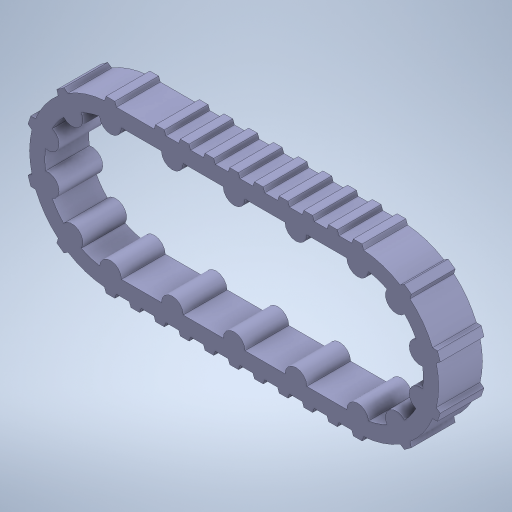
# Autodesk Inventor part: Guntas_Belt_New
Saved by Autodesk Inventor 2024 (Build 280153000, 153)
## iProperties
Created: 2023-07-07
Part Number: Guntas_Belt_New
Material: Generic
Document SubType Name: Modeling
Designer: manas
Density: 1 g/cm^3
Appearance: Slate Blue
Author: manas
Autodesk Inventor part; units mm, degrees
ref_plane "YZ Plane" through (0, 0, 0) normal (1, 0, 0) x (0, 1, 0)
ref_plane "XZ Plane" through (0, 0, 0) normal (0, 1, 0) x (-1, 0, 0)
ref_plane "XY Plane" through (0, 0, 0) normal (0, 0, 1) x (1, 0, 0)
sketch "Sketch1" plane through (0, 0, 0) normal (0, 0, 1) x (1, 0, 0)
  arc A0 (0, 75) -> (0, -75) centre (0, 0) ccw
  arc A1 (0, 92.5) -> (0, -92.5) centre (0, 0) ccw
  circle A2 centre (0, 75) radius 12.5
  circle A3 centre (-44.0839, 60.6763) radius 12.5
  circle A4 centre (-71.3292, 23.1763) radius 12.5
  circle A5 centre (-71.3292, -23.1763) radius 12.5
  circle A6 centre (-44.0839, -60.6763) radius 12.5
  circle A7 centre (0, -75) radius 12.5
  line L0 (0, 97.5) -> (-5, 97.5)
  line L1 (0, 97.5) -> (5, 97.5)
  line L2 (-5, 97.5) -> (-6.914, 92.2412)
  line L3 (-5, 97.5) -> (0.5963, 97.5) construction
  line L4 (5, 97.5) -> (6.914, 92.2412)
  line L5 (-57.3091, 78.8792) -> (-61.3541, 75.9402)
  line L6 (-61.3541, 75.9402) -> (-56.8267, 79.2296) construction
  line L7 (-57.3091, 78.8792) -> (-53.264, 81.8181)
  line L8 (-53.264, 81.8181) -> (-48.6245, 78.6887)
  line L9 (-61.3541, 75.9402) -> (-59.8116, 70.5608)
  line L10 (-92.728, 30.1292) -> (-94.2731, 25.3739)
  line L11 (-94.2731, 25.3739) -> (-92.5438, 30.6962) construction
  line L12 (-92.728, 30.1292) -> (-91.1829, 34.8844)
  line L13 (-91.1829, 34.8844) -> (-85.5901, 35.0797)
  line L14 (-94.2731, 25.3739) -> (-89.8632, 21.9285)
  line L15 (-92.728, -30.1292) -> (-91.1829, -34.8844)
  line L16 (-91.1829, -34.8844) -> (-92.9123, -29.5621) construction
  line L17 (-92.728, -30.1292) -> (-94.2731, -25.3739)
  line L18 (-94.2731, -25.3739) -> (-89.8632, -21.9285)
  line L19 (-91.1829, -34.8844) -> (-85.5901, -35.0797)
  line L20 (-57.3091, -78.8792) -> (-53.264, -81.8181)
  line L21 (-53.264, -81.8181) -> (-57.7914, -78.5287) construction
  line L22 (-57.3091, -78.8792) -> (-61.3541, -75.9402)
  line L23 (-61.3541, -75.9402) -> (-59.8116, -70.5608)
  line L24 (-53.264, -81.8181) -> (-48.6245, -78.6887)
  line L25 (0, -97.5) -> (5, -97.5)
  line L26 (5, -97.5) -> (-0.5963, -97.5) construction
  line L27 (0, -97.5) -> (-5, -97.5)
  line L28 (-5, -97.5) -> (-6.914, -92.2412)
  line L29 (5, -97.5) -> (6.914, -92.2412)
  line L30 (0, 92.5) -> (141.25, 92.5)
  line L31 (0, -92.5) -> (141.25, -92.5)
  line L32 (0, -92.5) -> (141.25, -92.5) construction
  line L33 (0, 75) -> (141.25, 75)
  line L34 (0, -75) -> (141.25, -75)
  line L35 (28.25, 97.5) -> (33.25, 97.5)
  line L36 (28.25, 97.5) -> (23.25, 97.5)
  line L37 (33.25, 97.5) -> (35.0699, 92.5)
  line L38 (23.25, 97.5) -> (21.4301, 92.5)
  line L39 (56.5, 97.5) -> (61.5, 97.5)
  line L40 (56.5, 97.5) -> (51.5, 97.5)
  line L41 (61.5, 97.5) -> (63.3199, 92.5)
  line L42 (51.5, 97.5) -> (49.6801, 92.5)
  line L43 (84.75, 97.5) -> (89.75, 97.5)
  line L44 (84.75, 97.5) -> (79.75, 97.5)
  line L45 (89.75, 97.5) -> (91.5699, 92.5)
  line L46 (79.75, 97.5) -> (77.9301, 92.5)
  line L47 (113, 97.5) -> (118, 97.5)
  line L48 (113, 97.5) -> (108, 97.5)
  line L49 (118, 97.5) -> (119.8199, 92.5)
  line L50 (108, 97.5) -> (106.1801, 92.5)
  line L51 (141.25, 97.5) -> (146.25, 97.5)
  line L52 (141.25, 97.5) -> (136.25, 97.5)
  line L53 (146.25, 97.5) -> (148.0699, 92.5)
  line L54 (136.25, 97.5) -> (134.4301, 92.5)
  circle A8 centre (70.625, 75) radius 12.5
  circle A9 centre (141.25, 75) radius 12.5
  line L55 (141.25, 92.5) -> (141.25, -92.5) construction
  line L56 (0, -92.5) -> (141.25, -92.5)
  line L57 (0, -75) -> (141.25, -75)
  line L58 (28.25, -97.5) -> (33.25, -97.5)
  line L59 (28.25, -97.5) -> (23.25, -97.5)
  line L60 (33.25, -97.5) -> (35.0699, -92.5)
  line L61 (23.25, -97.5) -> (21.4301, -92.5)
  line L62 (56.5, -97.5) -> (61.5, -97.5)
  line L63 (56.5, -97.5) -> (51.5, -97.5)
  line L64 (61.5, -97.5) -> (63.3199, -92.5)
  line L65 (51.5, -97.5) -> (49.6801, -92.5)
  line L66 (84.75, -97.5) -> (89.75, -97.5)
  line L67 (84.75, -97.5) -> (79.75, -97.5)
  line L68 (89.75, -97.5) -> (91.5699, -92.5)
  line L69 (79.75, -97.5) -> (77.9301, -92.5)
  line L70 (113, -97.5) -> (118, -97.5)
  line L71 (113, -97.5) -> (108, -97.5)
  line L72 (118, -97.5) -> (119.8199, -92.5)
  line L73 (108, -97.5) -> (106.1801, -92.5)
  line L74 (141.25, -97.5) -> (146.25, -97.5)
  line L75 (141.25, -97.5) -> (136.25, -97.5)
  line L76 (146.25, -97.5) -> (148.0699, -92.5)
  line L77 (136.25, -97.5) -> (134.4301, -92.5)
  circle A10 centre (70.625, -75) radius 12.5
  circle A11 centre (141.25, -75) radius 12.5
  line L78 (141.25, -92.5) -> (141.25, 92.5) construction
  arc A12 (282.5, -75) -> (282.5, 75) centre (282.5, 0) ccw
  arc A13 (282.5, -92.5) -> (282.5, 92.5) centre (282.5, 0) ccw
  circle A14 centre (282.5, 75) radius 12.5
  circle A15 centre (326.5839, 60.6763) radius 12.5
  circle A16 centre (353.8292, 23.1763) radius 12.5
  circle A17 centre (353.8292, -23.1763) radius 12.5
  circle A18 centre (326.5839, -60.6763) radius 12.5
  circle A19 centre (282.5, -75) radius 12.5
  line L79 (282.5, 97.5) -> (287.5, 97.5)
  line L80 (282.5, 97.5) -> (277.5, 97.5)
  line L81 (287.5, 97.5) -> (289.414, 92.2412)
  line L82 (287.5, 97.5) -> (281.9037, 97.5) construction
  line L83 (277.5, 97.5) -> (275.586, 92.2412)
  line L84 (339.8091, 78.8792) -> (343.8541, 75.9402)
  line L85 (343.8541, 75.9402) -> (339.3267, 79.2296) construction
  line L86 (339.8091, 78.8792) -> (335.764, 81.8181)
  line L87 (335.764, 81.8181) -> (331.1245, 78.6887)
  line L88 (343.8541, 75.9402) -> (342.3116, 70.5608)
  line L89 (375.228, 30.1292) -> (376.7731, 25.3739)
  line L90 (376.7731, 25.3739) -> (375.0438, 30.6962) construction
  line L91 (375.228, 30.1292) -> (373.6829, 34.8844)
  line L92 (373.6829, 34.8844) -> (368.0901, 35.0797)
  line L93 (376.7731, 25.3739) -> (372.3632, 21.9285)
  line L94 (375.228, -30.1292) -> (373.6829, -34.8844)
  line L95 (373.6829, -34.8844) -> (375.4123, -29.5621) construction
  line L96 (375.228, -30.1292) -> (376.7731, -25.3739)
  line L97 (376.7731, -25.3739) -> (372.3632, -21.9285)
  line L98 (373.6829, -34.8844) -> (368.0901, -35.0797)
  line L99 (339.8091, -78.8792) -> (335.764, -81.8181)
  line L100 (335.764, -81.8181) -> (340.2914, -78.5287) construction
  line L101 (339.8091, -78.8792) -> (343.8541, -75.9402)
  line L102 (343.8541, -75.9402) -> (342.3116, -70.5608)
  line L103 (335.764, -81.8181) -> (331.1245, -78.6887)
  line L104 (282.5, -97.5) -> (277.5, -97.5)
  line L105 (277.5, -97.5) -> (283.0963, -97.5) construction
  line L106 (282.5, -97.5) -> (287.5, -97.5)
  line L107 (287.5, -97.5) -> (289.414, -92.2412)
  line L108 (277.5, -97.5) -> (275.586, -92.2412)
  line L109 (282.5, 92.5) -> (141.25, 92.5)
  line L110 (282.5, -92.5) -> (141.25, -92.5)
  line L111 (282.5, -92.5) -> (141.25, -92.5) construction
  line L112 (282.5, 75) -> (141.25, 75)
  line L113 (282.5, -75) -> (141.25, -75)
  line L114 (254.25, 97.5) -> (249.25, 97.5)
  line L115 (254.25, 97.5) -> (259.25, 97.5)
  line L116 (249.25, 97.5) -> (247.4301, 92.5)
  line L117 (259.25, 97.5) -> (261.0699, 92.5)
  line L118 (226, 97.5) -> (221, 97.5)
  line L119 (226, 97.5) -> (231, 97.5)
  line L120 (221, 97.5) -> (219.1801, 92.5)
  line L121 (231, 97.5) -> (232.8199, 92.5)
  line L122 (197.75, 97.5) -> (192.75, 97.5)
  line L123 (197.75, 97.5) -> (202.75, 97.5)
  line L124 (192.75, 97.5) -> (190.9301, 92.5)
  line L125 (202.75, 97.5) -> (204.5699, 92.5)
  line L126 (169.5, 97.5) -> (164.5, 97.5)
  line L127 (169.5, 97.5) -> (174.5, 97.5)
  line L128 (164.5, 97.5) -> (162.6801, 92.5)
  line L129 (174.5, 97.5) -> (176.3199, 92.5)
  line L130 (141.25, 97.5) -> (136.25, 97.5)
  line L131 (141.25, 97.5) -> (146.25, 97.5)
  line L132 (136.25, 97.5) -> (134.4301, 92.5)
  line L133 (146.25, 97.5) -> (148.0699, 92.5)
  circle A20 centre (211.875, 75) radius 12.5
  circle A21 centre (141.25, 75) radius 12.5
  line L134 (282.5, -75) -> (141.25, -75)
  circle A22 centre (211.875, -75) radius 12.5
  line L135 (197.75, -97.5) -> (192.75, -97.5)
  line L136 (197.75, -97.5) -> (202.75, -97.5)
  line L137 (202.75, -97.5) -> (204.5699, -92.5)
  line L138 (282.5, -92.5) -> (141.25, -92.5)
  line L139 (259.25, -97.5) -> (261.0699, -92.5)
  line L140 (254.25, -97.5) -> (259.25, -97.5)
  line L141 (254.25, -97.5) -> (249.25, -97.5)
  line L142 (249.25, -97.5) -> (247.4301, -92.5)
  line L143 (221, -97.5) -> (219.1801, -92.5)
  line L144 (226, -97.5) -> (221, -97.5)
  line L145 (231, -97.5) -> (232.8199, -92.5)
  line L146 (226, -97.5) -> (231, -97.5)
  line L147 (169.5, -97.5) -> (164.5, -97.5)
  line L148 (169.5, -97.5) -> (174.5, -97.5)
  line L149 (164.5, -97.5) -> (162.6801, -92.5)
  line L150 (174.5, -97.5) -> (176.3199, -92.5)
  line L151 (192.75, -97.5) -> (190.9301, -92.5)
  line L152 (146.25, -97.5) -> (148.0699, -92.5)
  line L153 (141.25, -97.5) -> (146.25, -97.5)
  line L154 (141.25, -97.5) -> (136.25, -97.5)
  line L155 (136.25, -97.5) -> (134.4301, -92.5)
  circle A23 centre (141.25, -75) radius 12.5
  point P0 (270, -75)
  point P1 (224.375, -75)
  point P2 (199.375, -75)
  point P3 (153.75, -75)
  point P4 (128.75, -75)
  point P5 (83.125, -75)
  point P6 (58.125, -75)
  point P7 (12.5, -75)
  point P8 (-12.4565, -73.9583)
  point P9 (-33.3941, -67.1553)
  point P10 (-53.5492, -52.5118)
  point P11 (-66.4893, -34.7012)
  point P12 (-74.1878, -11.0075)
  point P13 (-74.1878, 11.0075)
  point P14 (-66.4893, 34.7012)
  point P15 (-53.5492, 52.5118)
  point P16 (-33.3941, 67.1553)
  point P17 (-12.4565, 73.9583)
  point P18 (12.5, 75)
  point P19 (58.125, 75)
  point P20 (83.125, 75)
  point P21 (128.75, 75)
  point P22 (153.75, 75)
  point P23 (199.375, 75)
  point P24 (224.375, 75)
  point P25 (270, 75)
  point P26 (294.9565, 73.9583)
  point P27 (315.8941, 67.1553)
  point P28 (336.0492, 52.5118)
  point P29 (348.9893, 34.7012)
  point P30 (356.6878, 11.0075)
  point P31 (356.6878, -11.0075)
  point P32 (348.9893, -34.7012)
  point P33 (336.0492, -52.5118)
  point P34 (315.8941, -67.1553)
  point P35 (294.9565, -73.9583)
  point P36 (6.8199, 92.5)
  point P37 (6.8199, -92.5)
  point P38 (275.6801, -92.5)
  point P39 (275.6801, 92.5)
  dimension "d5" = 180
  dimension "d13" = 180
  dimension "d29" = 28.25
  dimension "d38" = 70.625
  constraints: 312 end point, 98 symmetric about line, 24 centre point, 12 horizontal, 10 point on circle, 4 coincident, 4 midpoint, 4 point on line, 2 equal length, 1 tangent, 117 other
  measures "d29" distance of L36.end L40.end
  measures "d38" distance of A8.centre A9.centre
extrude "Extrusion1" add sketch "Sketch1" along normal mid plane 50 contours L33 A2 A0 | A0 A2 L33 | A3 A0 | A0 A3 | A8 L33 | L33 A8 | A4 A0 | A0 A4 | A9 L112 L33 | L33 L112 A9 | A5 A0 | A0 A5 | A20 L112 | L112 A20 | A6 A0 | A0 A6 | L112 A12 A14 | A14 A12 L112 | A7 L34 A0 | A0 L34 A7 | A15 A12 | A12 A15 | A10 L34 | L34 A10 | A16 A12 | A12 A16 | A11 L113 L34 | L34 L113 A11 | A17 A12 | A12 A17 | A22 L113 | L113 A22 | A18 A12 | A12 A18 | L113 A12 A19 | A19 A12 L113 | L30 L109 A13 L110 L31 A1 | A1 L2 L0 L1 L4 L30 | A1 L9 L5 L7 L8 | A1 L14 L10 L12 L13 | L42 L40 L39 L41 L30 | A1 L19 L15 L17 L18 | L46 L44 L43 L45 L30 | A1 L24 L20 L22 L23 | L50 L48 L47 L49 L30 | A1 L31 L29 L25 L27 L28 | L54 L52 L51 L53 L109 L30 | L31 L60 L58 L59 L61 | L128 L126 L127 L129 L109 | L31 L64 L62 L63 L65 | L124 L122 L123 L125 L109 | L31 L68 L66 L67 L69 | L120 L118 L119 L121 L109 | L31 L72 L70 L71 L73 | L116 L114 L115 L117 L109 | L31 L110 L76 L74 L75 L77 | L83 L80 L79 L81 A13 L109 | L110 L150 L148 L147 L149 | L87 L86 L84 L88 A13 | L110 L137 L136 L135 L151 | L92 L91 L89 L93 A13 | L110 L145 L146 L144 L143 | L97 L96 L94 L98 A13 | L110 L139 L140 L141 L142 | L102 L101 L99 L103 A13 | L110 A13 L107 L106 L104 L108
body "Solid1"
